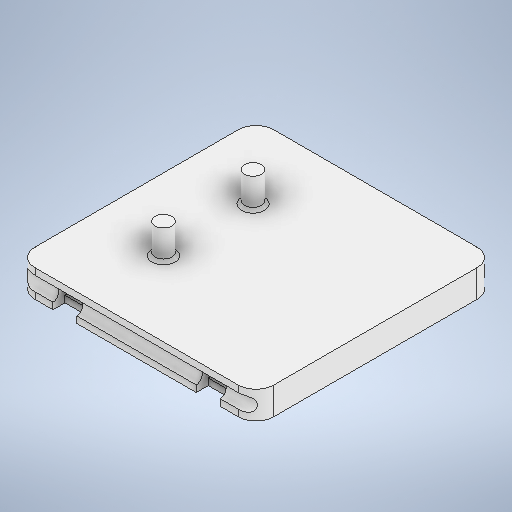
# Autodesk Inventor part: IMU_mount_baseplate
Saved by Autodesk Inventor 2025.2 (Build 292293000, 293)
## iProperties
Created: 2024-11-14
Part Number: IMU_mount_baseplate
Material: Generic
Document SubType Name: Modeling
Designer: matss
Density: 1 g/cm^3
Appearance: Default
Author: matss
Autodesk Inventor part; units mm, degrees
ref_plane "YZ Plane" through (0, 0, 0) normal (1, 0, 0) x (0, 1, 0)
ref_plane "XZ Plane" through (0, 0, 0) normal (0, 1, 0) x (-1, 0, 0)
sketch "Sketch1" plane through (0, 0, 0) normal (0, 1, 0) x (-1, 0, 0)
  line L0 (20, 20) -> (-20, 20)
  line L1 (-20, 20) -> (-20, -20)
  line L2 (-20, -20) -> (20, -20)
  line L3 (20, -20) -> (20, 20)
  circle A0 centre (10.5, 10.5) radius 4.25
  circle A1 centre (10.5, -10.5) radius 4.25
  circle A2 centre (-10.5, -10.5) radius 4.25
  circle A3 centre (-10.5, 10.5) radius 4.25
  line L4 (20, 0) -> (-20, 0) construction
  line L5 (0, 20) -> (0, -20) construction
  point P0 (0, 0)
  dimension "d0" = 40
  dimension "d1" = 40
  dimension "d2" = 8.5
  dimension "d3" = 21
  dimension "d4" = 21
  constraints: 12 end point, 4 centre point, 4 midpoint, 3 equal radius, 2 parallel, 1 horizontal, 1 horizontal alignment, 1 perpendicular, 1 vertical alignment, 3 other
  measures "d0" distance of L2.end L0.start
  measures "d1" distance of L0.start L0.end
  measures "d2" diameter of A0
  measures "d3" distance of A1.centre A0.centre
  measures "d4" distance of A3.centre A0.centre
extrude "Extrusion2" add sketch "Sketch1" along normal blind 2
sketch "Sketch2" plane through (0, 0, 0) normal (0, -1, 0) x (1, 0, 0)
  line L0 (20, 20) -> (20, -20) projected
  line L1 (-20, 20) -> (20, 20) projected
  line L2 (-20, -20) -> (-20, 20) projected
  line L3 (20, -20) -> (-20, -20) projected
  point P0 (0, 0)
extrude "Extrusion3" add sketch "Sketch2" along normal blind 0.6
sketch "Sketch3" plane through (0, 2, 0) normal (0, 1, 0) x (1, 0, 0)
  line L0 (-20, 20) -> (-20, -20) projected
  line L1 (-20, -20) -> (20, -20) projected
  line L2 (20, -20) -> (20, 20) projected
  line L3 (20, 20) -> (-20, 20) projected
  point P0 (0, 0)
extrude "Extrusion4" add sketch "Sketch3" along normal blind 2
fillet "Fillet1" radius 3 4 edges at (-20, 1.7, 20) (-20, 1.7, -20) (20, 1.7, 20) (20, 1.7, -20)
ref_plane "Arbeitsebene1" through (-17, 4, 20) normal (1, 0, 0) x (0, -1, 0)
sketch "Skizze5" plane through (-17, 4, 20) normal (1, 0, 0) x (0, -1, 0)
  line L0 (0, 0) -> (4.6, 0) construction
  line L1 (0, 0) -> (0, 3) construction
  line L2 (0.7, 0) -> (3.5, 0) construction
  line L3 (6.1491, 20) -> (-1.642, 20) construction
  line L4 (0, 40) -> (4.6, 40) construction
  line L5 (0.7, 40) -> (3.5, 40) construction
  line L6 (2.3, 0) -> (2.3, 4.6722) construction
  ellipse E0 centre (2.3, 0) end of major axis (3.5, 0) minor radius 1
  line L7 (1.1, 0) -> (3.5, 0)
  line L8 (0, 40) -> (4.6, 40) construction
  line L9 (0.7, 40) -> (3.5, 40) construction
  ellipse E1 centre (2.3, 40) end of major axis (3.5, 40) minor radius 1
  line L10 (1.1, 40) -> (3.5, 40)
  point P0 (4, 20)
  point P1 (2.3, 1)
  dimension "d22" = 2.3
  dimension "d23" = 1.2
  dimension "d28" = 1
  constraints: 18 end point, 9 point on line, 6 symmetric about line, 3 horizontal, 2 collinear, 2 midpoint, 1 coincident, 1 vertical, 9 other
  measures "d22" distance from line of L1 L6.start
  measures "d23" distance of L6.start L2.end
  measures "d28" distance of point (2.3, 0) point (2.3, 1)
extrude "Extrusion7" cut sketch "Skizze5" along normal blind 37 and the other way blind 5 contours L7 E0 | E1 L10 picked at (2.3176, 0.333) picked at (2.2824, 39.667)
sketch "Skizze6" plane through (0, -0.6, 0) normal (0, -1, 0) x (1, 0, 0)
  line L0 (17, 20) -> (-17, 20) projected
  line L1 (-20, 17) -> (-20, -17) construction
  line L2 (-14, 20) -> (-14, 16.5)
  line L3 (-14, 20) -> (-10, 20)
  line L4 (0, 16.6905) -> (0, 25.5183)
  line L5 (7.2129, 0) -> (-7.9382, 0)
  line L6 (-17, 20) -> (17, 20)
  line L7 (14, 20) -> (10, 20)
  line L8 (17, -20) -> (-17, -20)
  line L9 (-14, 16.5) -> (-10, 16.5)
  line L10 (-10, 16.5) -> (-10, 20)
  line L11 (-17, -20) -> (17, -20) projected
  line L12 (14, 20) -> (14, 16.5)
  line L13 (14, 16.5) -> (10, 16.5)
  line L14 (10, 16.5) -> (10, 20)
  line L15 (-14, -20) -> (-14, -16.5)
  line L16 (-14, -16.5) -> (-10, -16.5)
  line L17 (-10, -16.5) -> (-10, -20)
  line L18 (10, -16.5) -> (10, -20)
  line L19 (14, -16.5) -> (10, -16.5)
  line L20 (14, -20) -> (14, -16.5)
  point P0 (0, 0)
  point P1 (-12, 20)
  dimension "d34" = 8
  dimension "d35" = 2
  dimension "d41" = 3.5
  dimension "d42" = 4
  constraints: 36 end point, 17 symmetric about line, 6 point on line, 2 vertical, 1 collinear, 1 horizontal, 1 parallel, 1 perpendicular
  measures "d34" distance from line of L1 point (-12, 20)
  measures "d35" distance from line of point (-12, 20) L2
  measures "d41" distance of L2.start L2.end
  measures "d42" distance between parallel lines of L10 L2
extrude "Extrusion8" cut sketch "Skizze6" against normal blind 3.3
sketch "Skizze8" plane through (0, -0.6, 0) normal (0, -1, 0) x (1, 0, 0)
  line L0 (-10, 20) -> (-10, 16.5) projected
  line L1 (-10, 16.5) -> (-14, 16.5) projected
  line L2 (-14, -20) -> (-14, -16.5) projected
  line L3 (-14, -16.5) -> (-10, -16.5) projected
  line L4 (-10, -16.5) -> (-10, -20) projected
  line L5 (-10, -20) -> (10, -20) projected
  line L6 (10, -20) -> (10, -16.5) projected
  line L7 (10, -16.5) -> (14, -16.5) projected
  line L8 (14, -16.5) -> (14, -20) projected
  line L9 (14, -20) -> (17, -20) projected
  arc A0 (17, -20) -> (20, -17) centre (17, -17) ccw projected
  line L10 (20, -17) -> (20, 17) projected
  arc A1 (20, 17) -> (17, 20) centre (17, 17) ccw projected
  line L11 (17, 20) -> (14, 20) projected
  line L12 (14, 20) -> (14, 16.5) projected
  line L13 (14, 16.5) -> (10, 16.5) projected
  line L14 (10, 16.5) -> (10, 20) projected
  line L15 (10, 20) -> (-10, 20) projected
  line L16 (-10, 20) -> (-10, 16.5) projected
  line L17 (-10, 16.5) -> (-14, 16.5) projected
  line L18 (-14, 16.5) -> (-14, 20) projected
  line L19 (-14, 20) -> (-17, 20) projected
  arc A2 (-17, 20) -> (-20, 17) centre (-17, 17) ccw projected
  line L20 (-20, 17) -> (-20, -17) projected
  arc A3 (-20, -17) -> (-17, -20) centre (-17, -17) ccw projected
  line L21 (-17, -20) -> (-14, -20) projected
  line L22 (0, 16.7549) -> (0, 9.0333)
  line L23 (12, 0) -> (-14, 0)
  line L24 (-10, 16.5) -> (-14, 16.5)
  line L25 (-14, 16.5) -> (-14, 18)
  line L26 (-14, 18) -> (-10, 18)
  line L27 (-10, 18) -> (-10, 16.5)
  line L28 (10, 20) -> (10, 16.5)
  line L29 (10, 16.5) -> (14, 16.5)
  line L30 (14, 16.5) -> (14, 18)
  line L31 (14, 18) -> (10, 18)
  line L32 (10, 18) -> (10, 16.5)
  line L33 (-14, -18) -> (-10, -18)
  line L34 (14, -18) -> (10, -18)
  point P0 (0, 0)
  dimension "d47" = 1.5
  constraints: 26 end point, 11 symmetric about line, 2 horizontal, 2 parallel, 1 perpendicular, 1 point on line, 1 vertical
  measures "d47" distance between parallel lines of L26 L1
extrude "Extrusion10" add sketch "Skizze8" against normal blind 1.1 contours L0 L1 L18 L26 | L31 L12 L13 L14 | L2 L3 L4 L33 | L34 L6 L7 L8
sketch "Skizze9" plane through (0, 4, 0) normal (0, 1, 0) x (1, 0, 0)
  line L0 (-20, 17) -> (-20, -17) projected
  circle A0 centre (-8, -7.5) radius 1.4
  line L1 (-2.4635, 0) -> (-12.5282, 0) construction
  circle A1 centre (-8, 7.5) radius 1.4
  point P0 (0, 0)
  dimension "d55" = 7.5
  dimension "d56" = 12
  dimension "d57" = 2.8
  constraints: 2 centre point, 2 end point, 1 coincident, 1 horizontal, 1 symmetric about line, 1 other
  measures "d55" vertical distance of point (0, 0) point (-8, -7.5)
  measures "d56" distance from line of L0 point (-8, -7.5)
  measures "d57" diameter of A0
extrude "Extrusion11" add sketch "Skizze9" along normal blind 5
chamfer "Fasen2" distance 0.5 angle 45 2 edges at (-9.4, 4, -7.5) (-9.4, 4, 7.5)
body "Solid2"
